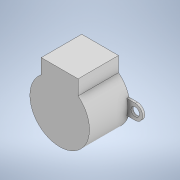
# Autodesk Inventor part: Stepper
Saved by Autodesk Inventor 2021 (Build 250183000, 183)
## iProperties
Created: 2023-12-28
Part Number: Stepper
Material: Generic
Document SubType Name: Modeling
Designer: maxsm
Density: 1 g/cm^3
Appearance: Default
Author: maxsm
Autodesk Inventor part; units mm, degrees
ref_plane "YZ Plane" through (0, 0, 0) normal (1, 0, 0) x (0, 1, 0)
ref_plane "XZ Plane" through (0, 0, 0) normal (0, 1, 0) x (-1, 0, 0)
ref_plane "XY Plane" through (0, 0, 0) normal (0, 0, 1) x (1, 0, 0)
sketch "Sketch1" plane through (0, 0, 0) normal (0, 0, 1) x (1, 0, 0)
  circle A0 centre (0, 0) radius 14
  dimension "d0" = 28
  constraints: 1 centre point, 1 coincident
  measures "d0" diameter of A0
extrude "Extrusion1" add sketch "Sketch1" along normal blind 19
sketch "Sketch2" plane through (0, 0, 0) normal (0, 0, 1) x (1, 0, 0)
  circle A0 centre (0, 0) radius 14 projected
  line L0 (-8.65, 18) -> (8.65, 18)
  line L1 (8.65, 18) -> (8.65, 0)
  line L2 (8.65, 0) -> (-8.65, 0)
  line L3 (-8.65, 0) -> (-8.65, 18)
  line L4 (-8.65, 18) -> (8.65, 0) construction
  line L5 (8.65, 18) -> (-8.65, 0) construction
  point P0 (0, 9)
  point P1 (0, 0)
  point P2 (0, 9)
  point P3 (0, 9)
  point P4 (0, -14)
  point P5 (-8.65, 11.0081)
  point P6 (8.65, 11.0081)
  dimension "d3" = 17.3
  dimension "d4" = 32
  constraints: 12 end point, 6 midpoint, 3 vertical alignment, 2 parallel, 1 horizontal, 1 perpendicular, 2 other
  measures "d3" distance between parallel lines of L1 L3
  measures "d4" distance from line of point (0, -14) L0
extrude "Extrusion2" add sketch "Sketch2" along normal blind 19 contours A0 L3 L0 L1
sketch "Sketch3" plane through (0, 0, 0) normal (0, 0, 1) x (1, 0, 0)
  line L0 (-8.65, 18) -> (8.65, 18) projected
  line L1 (8.65, 18) -> (8.65, 11.0081) projected
  arc A0 (-8.65, 11.0081) -> (8.65, 11.0081) centre (0, 0) ccw projected
  line L2 (-8.65, 11.0081) -> (-8.65, 18) projected
  line L3 (-21, 0) -> (0, 0) construction
  line L4 (-17.5, -3.5) -> (-3.5, -3.5)
  line L5 (-3.5, 3.5) -> (-17.5, 3.5)
  arc A1 (-17.5, 3.5) -> (-17.5, -3.5) centre (-17.5, 0) ccw
  arc A2 (-3.5, -3.5) -> (-3.5, 3.5) centre (-3.5, 0) ccw
  circle A3 centre (-17.5, 0) radius 2
  point P0 (-10.5, 0)
  point P1 (-13.5554, -3.5)
  point P2 (-13.5554, 3.5)
  dimension "d7" = 21
  dimension "d8" = 7
  dimension "d9" = 4
  constraints: 8 end point, 6 point on circle, 4 tangent, 3 centre point, 2 point on line, 1 coincident, 1 horizontal, 1 midpoint, 1 parallel
  measures "d7" distance of point (0, 0) L3.start
  measures "d8" distance between parallel lines of L4 L5
  measures "d9" diameter of A3
extrude "Extrusion3" add sketch "Sketch3" along normal blind 1 contours A0 L4 A1 L5
mirror "Mirror1" about plane through (0, 0, 0) normal (1, 0, 0) of "Extrusion3"
sketch "Sketch4" plane through (0, 0, 0) normal (0, 0, -1) x (-1, 0, 0)
  circle A0 centre (0, -7.25) radius 4.75
  line L0 (-8.65, 18) -> (8.65, 18) projected
  point P0 (0, 0)
  point P1 (0, -2.5)
  point P2 (0, -2.5)
  point P3 (0, 0)
  dimension "d12" = 9.5
  dimension "d13" = 20.5
  constraints: 3 vertical alignment, 2 coincident, 2 other
  measures "d13" distance from line of L0 point (0, -2.5)
extrude "Extrusion4" add sketch "Sketch4" along normal blind 1.5
sketch "Sketch5" plane through (0, -7.25, -1.5) normal (0, 0, -1) x (-1, 0, 0)
  circle A0 centre (0, 0) radius 2.5
  circle A1 centre (0, 0) radius 4.75 projected
  point P0 (0, 7.25)
  dimension "d16" = 5
  constraints: 1 centre point, 1 concentric
  measures "d16" diameter of A0
extrude "Extrusion5" add sketch "Sketch5" along normal blind 8 contours A0
body "Solid1"
